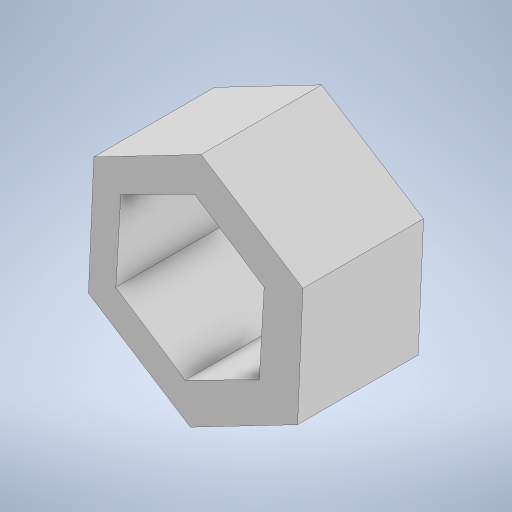
# Autodesk Inventor part: bolt
Saved by Autodesk Inventor 2023 (Build 270158000, 158)
## iProperties
Created: 2022-06-19
Part Number: bolt
Material: Generic
Document SubType Name: Modeling
Designer: ADITYA CHINAGUDI
Density: 1 g/cm^3
Appearance: Default
Author: ADITYA CHINAGUDI
Autodesk Inventor part; units mm, degrees
ref_plane "YZ Plane" through (0, 0, 0) normal (1, 0, 0) x (0, 1, 0)
ref_plane "XZ Plane" through (0, 0, 0) normal (0, 1, 0) x (-1, 0, 0)
ref_plane "XY Plane" through (0, 0, 0) normal (0, 0, 1) x (1, 0, 0)
sketch "Sketch1" plane through (0, 0, 0) normal (0, 0, 1) x (1, 0, 0)
  line L0 (-3.9091, 4.1274) -> (-6.5752, 2.7416)
  line L1 (-6.5752, 2.7416) -> (-9.1085, 4.3576)
  line L2 (-9.1085, 4.3576) -> (-8.9756, 7.3595)
  line L3 (-8.9756, 7.3595) -> (-6.3094, 8.7454)
  line L4 (-6.3094, 8.7454) -> (-3.7762, 7.1293)
  line L5 (-3.7762, 7.1293) -> (-3.9091, 4.1274)
  point P0 (0, 0)
  point P1 (-6.4423, 5.7435)
  constraints: 12 end point, 13 other
extrude "Extrusion1" add sketch "Sketch1" along normal blind 3
sketch "Sketch2" plane through (0, 0, 3) normal (0, 0, 1) x (1, 0, 0)
  line L0 (-6.7044, 3.6907) -> (-8.4267, 4.8255)
  line L1 (-8.4267, 4.8255) -> (-8.3051, 6.8846)
  line L2 (-8.3051, 6.8846) -> (-6.4611, 7.8087)
  line L3 (-6.4611, 7.8087) -> (-4.7388, 6.6739)
  line L4 (-4.7388, 6.6739) -> (-4.8604, 4.6149)
  line L5 (-4.8604, 4.6149) -> (-6.7044, 3.6907)
  line L6 (-8.9756, 7.3595) -> (-9.1085, 4.3576) projected
  point P0 (0, 0)
  point P1 (-6.5827, 5.7497)
  point P2 (-9.042, 5.8586)
  dimension "d2" = 2.4617
  constraints: 12 end point, 1 midpoint, 13 other
  measures "d2" distance of point (-9.042, 5.859) point (-6.583, 5.75)
extrude "Extrusion2" cut sketch "Sketch2" against normal blind 3
body "Solid1"
